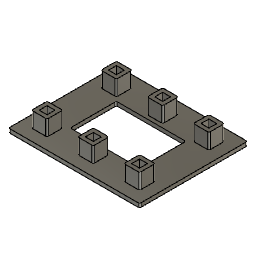
Project Stand Base Plate v7 (Autodesk Fusion 360 design; units mm, degrees)
Autodesk Fusion 360 part; units mm, degrees
sketch "Sketch1" plane through (0, 0, 0) normal (0, 0, 1) x (1, 0, 0)
  line L0 (-17.3001, 65.9212) -> (152.6999, 65.9212)
  line L1 (152.6999, 65.9212) -> (152.6999, -74.0788)
  line L2 (152.6999, -74.0788) -> (-17.3001, -74.0788)
  line L3 (-17.3001, -74.0788) -> (-17.3001, 65.9212)
  dimension "d1" = 140
  dimension "d2" = 170
  constraint horizontal L0
  constraint vertical L1
  constraint horizontal L2
  constraint vertical L3
  measures "d1" distance of L0 L2
  measures "d2" distance of L1 L3
extrude "Extrude1" add sketch "Sketch1" along normal blind 5
sketch "Sketch10" plane through (0, 0, 5) normal (0, 0, 1) x (-1, 0, 0)
  line L0 (17.3001, 74.0788) -> (-152.6999, 74.0788)
  line L1 (-152.6999, 74.0788) -> (-152.6999, -65.9212)
  line L2 (-152.6999, -65.9212) -> (17.3001, -65.9212)
  line L3 (17.3001, -65.9212) -> (17.3001, 74.0788)
  line L4 (-7.6999, -40.9212) -> (-127.6999, -40.9212)
  line L5 (-127.6999, -40.9212) -> (-127.6999, 49.0788)
  line L6 (-127.6999, 49.0788) -> (-7.6999, 49.0788)
  line L7 (-7.6999, 49.0788) -> (-7.6999, -40.9212)
  line L8 (17.3001, -65.9212) -> (-152.6999, -65.9212)
  line L9 (-152.6999, 74.0788) -> (17.3001, 74.0788)
  line L10 (17.3001, 74.0788) -> (17.3001, -65.9212)
  line L11 (-152.6999, -65.9212) -> (-152.6999, 74.0788)
  line L12 (-2.5999, -46.0212) -> (-12.7999, -46.0212)
  line L13 (-12.7999, -46.0212) -> (-12.7999, -35.8212)
  line L14 (-12.7999, -35.8212) -> (-2.5999, -35.8212)
  line L15 (-2.5999, -35.8212) -> (-2.5999, -46.0212)
  line L16 (-122.5999, -46.0212) -> (-132.7999, -46.0212)
  line L17 (-132.7999, -46.0212) -> (-132.7999, -35.8212)
  line L18 (-132.7999, -35.8212) -> (-122.5999, -35.8212)
  line L19 (-122.5999, -35.8212) -> (-122.5999, -46.0212)
  line L20 (-62.5999, -46.0212) -> (-72.7999, -46.0212)
  line L21 (-72.7999, -46.0212) -> (-72.7999, -35.8212)
  line L22 (-72.7999, -35.8212) -> (-62.5999, -35.8212)
  line L23 (-62.5999, -35.8212) -> (-62.5999, -46.0212)
  line L24 (-2.5999, 43.9788) -> (-12.7999, 43.9788)
  line L25 (-12.7999, 43.9788) -> (-12.7999, 54.1788)
  line L26 (-12.7999, 54.1788) -> (-2.5999, 54.1788)
  line L27 (-2.5999, 54.1788) -> (-2.5999, 43.9788)
  line L28 (-122.5999, 43.9788) -> (-132.7999, 43.9788)
  line L29 (-132.7999, 43.9788) -> (-132.7999, 54.1788)
  line L30 (-132.7999, 54.1788) -> (-122.5999, 54.1788)
  line L31 (-122.5999, 54.1788) -> (-122.5999, 43.9788)
  line L32 (-62.5999, 43.9788) -> (-72.7999, 43.9788)
  line L33 (-72.7999, 43.9788) -> (-72.7999, 54.1788)
  line L34 (-72.7999, 54.1788) -> (-62.5999, 54.1788)
  line L35 (-62.5999, 54.1788) -> (-62.5999, 43.9788)
  line L36 (-22.6999, -25.9212) -> (-112.6999, -25.9212)
  line L37 (-112.6999, -25.9212) -> (-112.6999, 34.0788)
  line L38 (-112.6999, 34.0788) -> (-22.6999, 34.0788)
  line L39 (-22.6999, 34.0788) -> (-22.6999, -25.9212)
  line L40 (2.4001, -51.0212) -> (-17.7999, -51.0212)
  line L41 (-17.7999, -51.0212) -> (-17.7999, -30.8212)
  line L42 (-17.7999, -30.8212) -> (2.4001, -30.8212)
  line L43 (2.4001, -30.8212) -> (2.4001, -51.0212)
  line L44 (-57.5999, -51.0212) -> (-77.7999, -51.0212)
  line L45 (-77.7999, -51.0212) -> (-77.7999, -30.8212)
  line L46 (-77.7999, -30.8212) -> (-57.5999, -30.8212)
  line L47 (-57.5999, -30.8212) -> (-57.5999, -51.0212)
  line L48 (-117.5999, -51.0212) -> (-137.7999, -51.0212)
  line L49 (-137.7999, -51.0212) -> (-137.7999, -30.8212)
  line L50 (-137.7999, -30.8212) -> (-117.5999, -30.8212)
  line L51 (-117.5999, -30.8212) -> (-117.5999, -51.0212)
  line L52 (-117.5999, 38.9788) -> (-137.7999, 38.9788)
  line L53 (-137.7999, 38.9788) -> (-137.7999, 59.1788)
  line L54 (-137.7999, 59.1788) -> (-117.5999, 59.1788)
  line L55 (-117.5999, 59.1788) -> (-117.5999, 38.9788)
  line L56 (-57.5999, 38.9788) -> (-77.7999, 38.9788)
  line L57 (-77.7999, 38.9788) -> (-77.7999, 59.1788)
  line L58 (-77.7999, 59.1788) -> (-57.5999, 59.1788)
  line L59 (-57.5999, 59.1788) -> (-57.5999, 38.9788)
  line L60 (2.4001, 38.9788) -> (-17.7999, 38.9788)
  line L61 (-17.7999, 38.9788) -> (-17.7999, 59.1788)
  line L62 (-17.7999, 59.1788) -> (2.4001, 59.1788)
  line L63 (2.4001, 59.1788) -> (2.4001, 38.9788)
  dimension "d65" = 25
  dimension "d66" = 25
  dimension "d67" = 25
  dimension "d68" = 25
  dimension "d69" = 5.1
  dimension "d70" = 5.1
  dimension "d71" = 5.1
  dimension "d72" = 5.1
  dimension "d73" = 5.1
  dimension "d74" = 5.1
  dimension "d75" = 5.1
  dimension "d76" = 5.1
  dimension "d77" = 109.8
  dimension "d78" = 19.9
  dimension "d79" = 19.9
  dimension "d80" = 49.8
  dimension "d81" = 49.8
  dimension "d82" = 5.1
  dimension "d83" = 5.1
  dimension "d84" = 5.1
  dimension "d85" = 5.1
  dimension "d86" = 5.1
  dimension "d87" = 5.1
  dimension "d88" = 5.1
  dimension "d89" = 5.1
  dimension "d90" = 5.1
  dimension "d91" = 5.1
  dimension "d92" = 49.8
  dimension "d93" = 49.8
  dimension "d94" = 5.1
  dimension "d95" = 5.1
  dimension "d96" = 15
  dimension "d97" = 15
  dimension "d98" = 15
  dimension "d99" = 15
  dimension "d100" = 5
  dimension "d101" = 5
  dimension "d102" = 5
  dimension "d103" = 5
  dimension "d104" = 5
  dimension "d105" = 5
  dimension "d106" = 5
  dimension "d107" = 5
  dimension "d108" = 5
  dimension "d109" = 5
  dimension "d110" = 5
  dimension "d111" = 5
  dimension "d112" = 5
  dimension "d113" = 5
  dimension "d114" = 5
  dimension "d115" = 5
  dimension "d116" = 5
  dimension "d117" = 5
  dimension "d118" = 5
  dimension "d119" = 5
  dimension "d120" = 5
  dimension "d121" = 5
  dimension "d122" = 5
  dimension "d123" = 5
  constraint horizontal L4
  constraint vertical L5
  constraint horizontal L6
  constraint vertical L7
  constraint horizontal L12
  constraint vertical L13
  constraint horizontal L14
  constraint vertical L15
  constraint horizontal L16
  constraint vertical L17
  constraint horizontal L18
  constraint vertical L19
  constraint horizontal L20
  constraint vertical L21
  constraint horizontal L22
  constraint vertical L23
  constraint horizontal L24
  constraint vertical L25
  constraint horizontal L26
  constraint vertical L27
  constraint horizontal L28
  constraint vertical L29
  constraint horizontal L30
  constraint vertical L31
  constraint horizontal L32
  constraint vertical L33
  constraint horizontal L34
  constraint vertical L35
  constraint horizontal L36
  constraint vertical L37
  constraint horizontal L38
  constraint vertical L39
  constraint horizontal L40
  constraint vertical L41
  constraint horizontal L42
  constraint vertical L43
  constraint horizontal L44
  constraint vertical L45
  constraint horizontal L46
  constraint vertical L47
  constraint horizontal L48
  constraint vertical L49
  constraint horizontal L50
  constraint vertical L51
  constraint horizontal L52
  constraint vertical L53
  constraint horizontal L54
  constraint vertical L55
  constraint horizontal L56
  constraint vertical L57
  constraint horizontal L58
  constraint vertical L59
  constraint horizontal L60
  constraint vertical L61
  constraint horizontal L62
  constraint vertical L63
  measures "d65" distance of L4 L8
  measures "d66" distance of L6 L9
  measures "d67" distance of L7 L10
  measures "d68" distance of L5 L11
  measures "d69" distance of L4.start L12
  measures "d70" distance of L4.start L15
  measures "d71" distance of L4.start L13
  measures "d72" distance of L4.start L14
  measures "d73" distance of L4.end L16
  measures "d74" distance of L4.end L17
  measures "d75" distance of L4.end L18
  measures "d76" distance of L4.end L19
  measures "d77" distance of L13 L19
  measures "d78" distance of L8 L12
  measures "d79" distance of L10 L15
  measures "d80" distance of L13 L23
  measures "d81" distance of L19 L21
  measures "d82" distance of L4 L20
  measures "d83" distance of L4 L22
  measures "d84" distance of L6.end L24
  measures "d85" distance of L6.end L27
  measures "d86" distance of L6.end L25
  measures "d87" distance of L6.end L26
  measures "d88" distance of L5.end L28
  measures "d89" distance of L5.end L29
  measures "d90" distance of L5.end L30
  measures "d91" distance of L5.end L31
  measures "d92" distance of L25 L35
  measures "d93" distance of L31 L33
  measures "d94" distance of L6 L32
  measures "d95" distance of L6 L34
  measures "d96" distance of L4 L36
  measures "d97" distance of L7 L39
  measures "d98" distance of L5 L37
  measures "d99" distance of L6 L38
  measures "d100" distance of L12 L40
  measures "d101" distance of L13 L41
  measures "d102" distance of L14 L42
  measures "d103" distance of L15 L43
  measures "d104" distance of L22 L46
  measures "d105" distance of L21 L45
  measures "d106" distance of L20 L44
  measures "d107" distance of L23 L47
  measures "d108" distance of L16 L48
  measures "d109" distance of L19 L51
  measures "d110" distance of L18 L50
  measures "d111" distance of L17 L49
  measures "d112" distance of L28 L52
  measures "d113" distance of L29 L53
  measures "d114" distance of L30 L54
  measures "d115" distance of L31 L55
  measures "d116" distance of L32 L56
  measures "d117" distance of L33 L57
  measures "d118" distance of L34 L58
  measures "d119" distance of L35 L59
  measures "d120" distance of L25 L61
  measures "d121" distance of L24 L60
  measures "d122" distance of L27 L63
  measures "d123" distance of L26 L62
extrude "Extrude8" cut sketch "Sketch10" against normal blind 5 contours L36 L37 L38 L39
extrude "Extrude9" cut sketch "Sketch10" against normal blind 2.5 contours L4 L7 L12 L13 L14 L15 | L4 L7 L13 L14 | L4 L20 L21 L23 | L4 L21 L22 L23 | L6 L7 L24 L25 | L6 L7 L24 L25 L26 L27 | L6 L32 L33 L35 | L6 L33 L34 L35 | L4 L5 L16 L17 L18 L19 | L4 L5 L18 L19 | L5 L6 L28 L29 L30 L31 | L5 L6 L28 L31
extrude "Extrude10" add sketch "Sketch10" along normal blind 10 contours L4 L7 L12 L13 L14 L15 L40 L41 L42 L43 | L4 L7 L13 L14 L41 L42 | L4 L20 L21 L23 L44 L45 L47 | L4 L21 L22 L23 L45 L46 L47 | L6 L7 L24 L25 L60 L61 | L6 L7 L24 L25 L26 L27 L60 L61 L62 L63 | L6 L32 L33 L35 L56 L57 L59 | L6 L33 L34 L35 L57 L58 L59 | L4 L5 L16 L17 L18 L19 L48 L49 L50 L51 | L4 L5 L18 L19 L50 L51 | L5 L6 L28 L29 L30 L31 L52 L53 L54 L55 | L5 L6 L28 L31 L52 L55
fillet "Fillet1" radius 2 4 edges at (152.6999, -74.0788, 2.5) (152.6999, 65.9212, 2.5) (-17.3001, 65.9212, 2.5) (-17.3001, -74.0788, 2.5)
extrude "Extrude11" add 6 faces at (5.9999, 49.3545, 15) (76.1332, 39.2212, 15) (136.1332, 39.2212, 15) (136.1332, -50.7788, 15) (76.1332, -50.7788, 15) (5.9999, -40.6455, 15) along direction (0, 0, 1) blind 10
fillet "Fillet2" radius 2 24 edges at (17.7999, 30.8212, 15) (-2.4001, 30.8212, 15) (57.5999, 30.8212, 15) (77.7999, 30.8212, 15) (117.5999, 30.8212, 15) (137.7999, 30.8212, 15) (57.5999, -59.1788, 15) (77.7999, -59.1788, 15) (17.7999, -59.1788, 15) (-2.4001, -59.1788, 15) (-2.4001, -38.9788, 15) (-2.4001, 51.0212, 15) (57.5999, 51.0212, 15) (117.5999, 51.0212, 15) (117.5999, -38.9788, 15) (117.5999, -59.1788, 15) (57.5999, -38.9788, 15) (77.7999, -38.9788, 15) (137.7999, -59.1788, 15) (137.7999, -38.9788, 15) (77.7999, 51.0212, 15) (137.7999, 51.0212, 15) (17.7999, 51.0212, 15) (17.7999, -38.9788, 15)
fillet "Fillet3" radius 2 4 edges at (22.6999, 25.9212, 2.5) (22.6999, -34.0788, 2.5) (112.6999, -34.0788, 2.5) (112.6999, 25.9212, 2.5)
